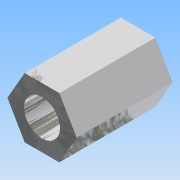
# Autodesk Inventor part: entretoise_8
Saved by Autodesk Inventor 2015 (Build 190159000, 159)
## iProperties
Created: 2016-04-17
Part Number: entretoise_8
Material: Générique
Document SubType Name: Modeling
Designer: Gregwar
Density: 1 g/cm^3
Appearance: Par défaut
Author: Gregwar
Autodesk Inventor part; units mm, degrees
ref_plane "YZ Plane" through (0, 0, 0) normal (1, 0, 0) x (0, 1, 0)
ref_plane "XZ Plane" through (0, 0, 0) normal (0, 1, 0) x (-1, 0, 0)
ref_plane "XY Plane" through (0, 0, 0) normal (0, 0, 1) x (1, 0, 0)
sketch "Esquisse1" plane through (0, 0, 0) normal (0, 1, 0) x (-1, 0, 0)
  line L0 (-1.4434, -2.5) -> (-2.8868, 0)
  line L1 (-2.8868, 0) -> (-1.4434, 2.5)
  line L2 (-1.4434, 2.5) -> (1.4434, 2.5)
  line L3 (1.4434, 2.5) -> (2.8868, 0)
  line L4 (2.8868, 0) -> (1.4434, -2.5)
  line L5 (1.4434, -2.5) -> (-1.4434, -2.5)
  circle A0 centre (0, 0) radius 1.5
  dimension "d0" = 3
  dimension "d1" = 5
  constraints: 12 end point, 2 coincident, 1 centre point, 1 horizontal, 13 other
  measures "d0" diameter of A0
  measures "d1" distance between parallel lines of L1 L4
extrude "Extrusion1" add sketch "Esquisse1" along normal blind 8
